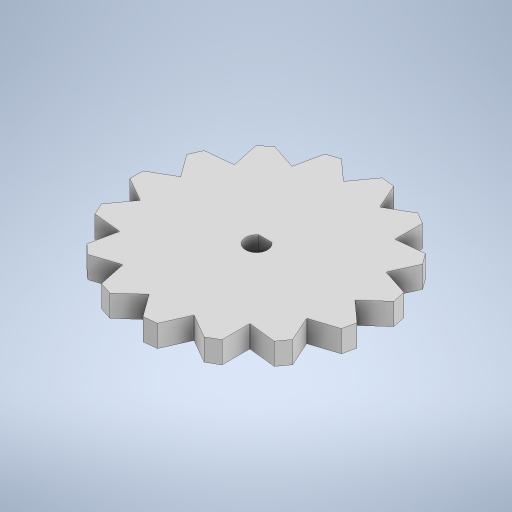
# Autodesk Inventor part: motor_gear
Saved by Autodesk Inventor 2023 (Build 270158000, 158)
## iProperties
Created: 2023-03-07
Part Number: motor_gear
Material: Generic
Document SubType Name: Modeling
Designer: caleb
Density: 1 g/cm^3
Appearance: Default
Author: caleb
Autodesk Inventor part; units mm, degrees
ref_plane "YZ Plane" through (0, 0, 0) normal (1, 0, 0) x (0, 1, 0)
ref_plane "XZ Plane" through (0, 0, 0) normal (0, 1, 0) x (-1, 0, 0)
ref_plane "XY Plane" through (0, 0, 0) normal (0, 0, 1) x (1, 0, 0)
sketch "Sketch1" plane through (0, 0, 0) normal (0, 1, 0) x (-1, 0, 0)
  circle A0 centre (0, 0) radius 22.5
  circle A1 centre (0, 0) radius 2.5
  line L0 (0, 2.5) -> (0, -2)
  line L1 (0, -2) -> (1.5, -2)
  line L2 (0, -2) -> (-1.5, -2)
  line L3 (22.4999, 0.0635) -> (29.9999, 0.0635)
  line L4 (27.4018, -1.4365) -> (22.0387, -4.5329)
  line L5 (27.4018, 1.5635) -> (22.0085, 4.6774)
  line L6 (29.9999, 0.0635) -> (36.2276, 0.0635) construction
  line L7 (27.4018, 1.5635) -> (27.4018, -1.4365)
  line L8 (25.6171, 9.833) -> (21.977, 4.8229)
  line L9 (24.3969, 12.5737) -> (25.6171, 9.833)
  line L10 (24.3969, 12.5737) -> (18.2033, 13.2247)
  line L11 (19.4029, 19.4023) -> (18.1154, 13.3448)
  line L12 (17.1735, 21.4097) -> (19.4029, 19.4023)
  line L13 (17.1735, 21.4097) -> (11.2506, 19.4853)
  line L14 (9.8338, 25.6168) -> (11.1214, 19.5593)
  line L15 (6.9806, 26.5438) -> (9.8338, 25.6168)
  line L16 (6.9806, 26.5438) -> (2.3525, 22.3767)
  line L17 (-1.4357, 27.4019) -> (2.2044, 22.3918)
  line L18 (-4.4192, 27.0883) -> (-1.4357, 27.4019)
  line L19 (-4.4192, 27.0883) -> (-6.9523, 21.399)
  line L20 (-12.4569, 24.4489) -> (-7.0937, 21.3525)
  line L21 (-15.055, 22.9489) -> (-12.4569, 24.4489)
  line L22 (-15.055, 22.9489) -> (-15.055, 16.7212)
  line L23 (-21.3242, 17.2685) -> (-15.1653, 16.6212)
  line L24 (-23.0876, 14.8415) -> (-21.3242, 17.2685)
  line L25 (-23.0876, 14.8415) -> (-20.5545, 9.1522)
  line L26 (-26.5044, 7.1023) -> (-20.6146, 9.0159)
  line L27 (-27.1281, 4.1678) -> (-26.5044, 7.1023)
  line L28 (-27.1281, 4.1678) -> (-22.5, 0.0006)
  line L29 (-27.1017, -4.2921) -> (-22.4995, -0.1482)
  line L30 (-26.478, -7.2265) -> (-27.1017, -4.2921)
  line L31 (-26.478, -7.2265) -> (-20.555, -9.151)
  line L32 (-23.0129, -14.9443) -> (-20.494, -9.2868)
  line L33 (-21.2495, -17.3713) -> (-23.0129, -14.9443)
  line L34 (-21.2495, -17.3713) -> (-15.0559, -16.7203)
  line L35 (-14.9449, -23.0124) -> (-14.9449, -16.8196)
  line L36 (-12.3469, -24.5124) -> (-14.9449, -23.0124)
  line L37 (-12.3469, -24.5124) -> (-6.9535, -21.3986)
  line L38 (-4.2929, -27.1016) -> (-6.8117, -21.4441)
  line L39 (-1.3093, -27.4152) -> (-4.2929, -27.1016)
  line L40 (-1.3093, -27.4152) -> (2.3513, -22.3768)
  line L41 (7.1015, -26.5046) -> (2.4993, -22.3608)
  line L42 (9.9546, -25.5775) -> (7.1015, -26.5046)
  line L43 (9.9546, -25.5775) -> (11.2494, -19.4859)
  line L44 (17.2679, -21.3247) -> (11.3781, -19.411)
  line L45 (19.4973, -19.3173) -> (17.2679, -21.3247)
  line L46 (19.4973, -19.3173) -> (18.2025, -13.2257)
  line L47 (24.4486, -12.4576) -> (18.2896, -13.1049)
  line L48 (25.6688, -9.717) -> (24.4486, -12.4576)
  line L49 (25.6688, -9.717) -> (22.0082, -4.6786)
  dimension "d0" = 45
  dimension "d1" = 5
  dimension "d2" = 4.5
  dimension "d3" = 7.5
  dimension "d4" = 30
  dimension "d5" = 150
  dimension "d6" = 3
  dimension "d7" = 3
  dimension "d24" = 360
  constraints: 100 end point, 3 horizontal, 3 point on circle, 3 point on line, 2 coincident, 1 centre point, 1 equal length, 1 vertical, 111 other
  measures "d1" diameter of A1
  measures "d2" distance of L0.start L0.end
  measures "d3" distance of L3.start L3.end
  measures "d4" angle of L3 L4
  measures "d5" angle of L6 L5
  measures "d6" distance of L5.start L3.end
  measures "d7" distance of L4.start L3.end
extrude "Extrusion1" add sketch "Sketch1" along normal blind 5 contours A0 | A0 L3 L7 L4 | A0 L5 L7 L3 | L49 L48 L47 A0 | A0 L10 L9 L8 | L46 L45 L44 A0 | A0 L13 L12 L11 | L43 L42 L41 A0 | A0 L16 L15 L14 | L40 L39 L38 A0 | A0 L19 L18 L17 | L37 L36 L35 A0 | A0 L22 L21 L20 | L34 L33 L32 A0 | A0 L25 L24 L23 | L31 L30 L29 A0 | A0 L28 L27 L26 | A1 L2 L1
equation "\"d7\" = d6"
body "Solid1"
